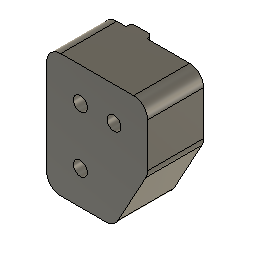
_cable chain mount plate.99133da1-0a92-4034-bb52-af1f1179e3d7 (Autodesk Fusion 360 design; units mm, degrees)
Autodesk Fusion 360 part; units mm, degrees
sketch "Sketch1" plane through (0, 0, 0) normal (0, 1, 0) x (1, 0, 0)
  circle A0 centre (0, 0) radius 2.5
  circle A1 centre (12, 0) radius 2.5
  line L0 (-12, -12) -> (24, -12)
  line L1 (24, -12) -> (24, 10)
  line L2 (24, 10) -> (12, 32)
  line L3 (12, 32) -> (-12, 32)
  line L4 (-12, 32) -> (-12, -12)
  line L5 (0, 0) -> (0, 32) construction
  circle A2 centre (0, 20) radius 2.5
  line L6 (0, 0) -> (0, 20) construction
  point P0 (0, 10)
  dimension "d1" = 5
  dimension "d3" = 12
  dimension "d5" = 12
  dimension "d6" = 20
  dimension "d7" = 12
  dimension "d8" = 12
  dimension "d9" = 12
  constraint coincident A0.centre L5.start
  constraint horizontal A0.centre A1.centre
  constraint horizontal L0
  constraint perpendicular L0 L1
  constraint perpendicular L1 L3
  constraint vertical L4
  constraint midpoint L3 L5.end
  constraint vertical L5
  constraint coincident L5 A2.centre
  constraint equal A0 A1
  constraint equal A0 A2
  constraint coincident A2.centre L6.end
  constraint midpoint L6 P0
  constraint horizontal L1.end P0
  measures "d1" diameter of A0
  measures "d3" distance of A0.centre A1.centre
  measures "d5" distance of A0.centre L4
  measures "d6" distance of A0.centre A2.centre
  measures "d7" distance of A0.centre L0
  measures "d8" distance of A1.centre L1
  measures "d9" distance of L3 A2.centre
extrude "Extrude1" add sketch "Sketch1" along normal blind 20
fillet "Fillet1" radius 5 5 edges at (-12, 10, 12) (24, 10, 12) (-12, 10, -32) (12, 10, -32) (24, 10, -10)
sketch "Sketch2" plane through (0, 20, 0) normal (0, 1, 0) x (-1, 0, 0)
  arc A0 (-24, -8.725) -> (-23.3895, -11.1193) centre (-19, -8.725) ccw
  line L0 (-23.3895, -11.1193) -> (-13.4213, -29.3943)
  arc A1 (-13.4213, -29.3943) -> (-9.0318, -32) centre (-9.0318, -27) ccw
  line L1 (-9.0318, -32) -> (7, -32)
  arc A2 (7, -32) -> (12, -27) centre (7, -27) ccw
  line L2 (12, -27) -> (12, 7)
  arc A3 (12, 7) -> (7, 12) centre (7, 7) ccw
  line L3 (7, 12) -> (-19, 12)
  arc A4 (-19, 12) -> (-24, 7) centre (-19, 7) ccw
  line L4 (-24, 7) -> (-24, -8.725)
  circle A5 centre (0, -20) radius 2.5
  circle A6 centre (0, 0) radius 2.5
  circle A7 centre (-12, 0) radius 2.5
  line L5 (0, 0) -> (0, -20) construction
  line L6 (-3.75, 12) -> (3.75, 12)
  line L7 (3.75, 12) -> (3.75, -32)
  line L8 (3.75, -32) -> (-3.75, -32)
  line L9 (-3.75, -32) -> (-3.75, 12)
  dimension "d15" = 7.5
  constraint coincident A6.centre L5.start
  constraint coincident A5.centre L5.end
  constraint horizontal L6
  constraint vertical L7
  constraint horizontal L8
  constraint vertical L9
  constraint coincident L1 L7.end
  constraint coincident L3 L6.start
  measures "d15" distance of L6.start L6.end
extrude "Extrude2" add sketch "Sketch2" along normal blind 2 contours L1 L3 L6 L7 L8 L9
chamfer "Chamfer1" distance 1 angle 45 2 edges at (3.75, 22, -10) (-3.75, 22, -10)
